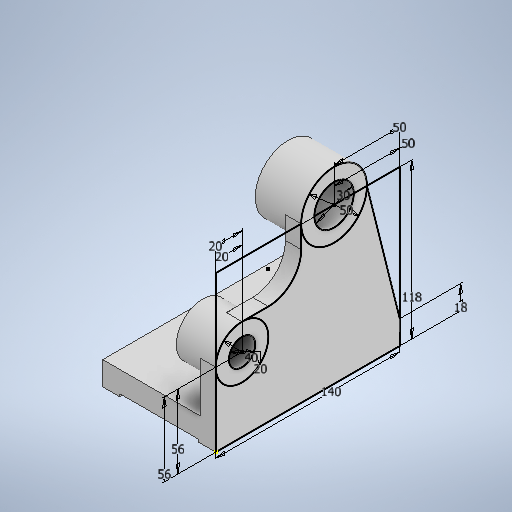
# Autodesk Inventor part: 3
Saved by Autodesk Inventor 2025.2 (Build 292293000, 293)
## iProperties
Created: 2024-12-04
Part Number: 3
Material: Generic
Document SubType Name: Modeling
Designer: hongquan
Density: 1 g/cm^3
Appearance: Default
Author: hongquan
Autodesk Inventor part; units mm, degrees
ref_plane "YZ Plane" through (0, 0, 0) normal (1, 0, 0) x (0, 1, 0)
ref_plane "XZ Plane" through (0, 0, 0) normal (0, 1, 0) x (-1, 0, 0)
ref_plane "XY Plane" through (0, 0, 0) normal (0, 0, 1) x (1, 0, 0)
sketch "Sketch1" plane through (0, 0, 0) normal (1, 0, 0) x (0, 1, 0)
  point P0 (0, 0)
sketch "Sketch2" plane through (0, 0, 0) normal (1, 0, 0) x (0, 1, 0)
  line L0 (0, 0) -> (118, 0)
  line L1 (118, 0) -> (118, -140)
  line L2 (118, -140) -> (0, -140)
  line L3 (0, -140) -> (0, 0)
  circle A0 centre (56, -20) radius 20
  circle A1 centre (56, -20) radius 10
  circle A2 centre (118, -90) radius 15
  circle A3 centre (118, -90) radius 25
  line L4 (118, -115) -> (18, -140)
  line L5 (101, -65) -> (118, -65)
  line L6 (76, -20) -> (76, -40)
  arc A4 (76, -40) -> (101, -65) centre (101, -40) ccw
  point P0 (56, 0)
  dimension "d2" = 40
  dimension "d0" = 140
  dimension "d1" = 118
  dimension "d3" = 20
  dimension "d4" = 30
  dimension "d5" = 50
  dimension "d6" = 56
  dimension "d7" = 56
  dimension "d8" = 20
  dimension "d9" = 20
  dimension "d10" = 50
  dimension "d11" = 50
  dimension "d12" = 18
  constraints: 14 end point, 4 centre point, 4 point on circle, 4 point on line, 3 tangent, 2 horizontal, 2 parallel, 1 perpendicular, 1 vertical, 4 other
  measures "d0" distance of L2.end L0.start
  measures "d1" distance of L1.end L2.end
  measures "d3" diameter of A1
  measures "d4" diameter of A2
  measures "d5" diameter of A3
  measures "d6" distance from line of L3 A1.centre
  measures "d7" distance from line of L3 point (56, -20)
  measures "d8" distance from line of L0 A1.centre
  measures "d9" distance from line of L0 point (56, -20)
  measures "d10" distance from line of L2 A2.centre
  measures "d11" distance from line of L2 A3.centre
  measures "d12" distance from line of L3 L4.end
sketch "Sketch3" plane through (0, 0, 0) normal (0, 0, 1) x (1, 0, 0)
  line L0 (0, 0) -> (-86, 0)
  line L1 (-86, 0) -> (-86, 18)
  line L2 (-86, 18) -> (0, 18)
  line L3 (0, 18) -> (0, 0)
  line L4 (-73, 2) -> (-13, 2)
  line L5 (-43, 18) -> (-43, 0)
  line L6 (-73, 2) -> (-73, 0)
  line L7 (-13, 2) -> (-13, 0)
  point P0 (-43, 2)
  dimension "d14" = 86
  dimension "d15" = 18
  dimension "d16" = 60
  dimension "d17" = 2
  constraints: 16 end point, 5 perpendicular, 3 midpoint, 3 point on line, 2 horizontal
  measures "d14" distance of L0.start L0.end
  measures "d15" distance of L0.end L1.end
  measures "d16" distance of L4.start L4.end
  measures "d17" distance between parallel lines of L0 L4
extrude "Extrusion1" add sketch "Sketch3" against normal blind 140 contours L0 L7 L4 L5 L2 L3 | L5 L4 L6 L0 L1 L2
extrude "Extrusion2" add sketch "Sketch2" against normal blind 12 contours L0 A0 L6 A4 L5 A3 L4 L2 L3
extrude "Extrusion3" add sketch "Sketch2" against normal blind 30 contours A0
extrude "Extrusion4" add sketch "Sketch2" against normal blind 35 contours A3 L1 A2 | L1 A2 A3
sketch "Sketch4" plane through (-73, 2, 0) normal (0, -1, 0) x (1, 0, 0)
  circle A0 centre (28.7142, -108.9689) radius 5
  circle A1 centre (33.7142, -71.4681) radius 5
  circle A2 centre (21.1452, -46.0088) radius 5
  line L0 (43, 0) -> (43, -40) projected
  circle A3 centre (43, -35.8595) radius 5
  point P0 (73, 0)
  dimension "d26" = 10
  dimension "d27" = 10
  dimension "d28" = 10
  dimension "d29" = 10
  constraints: 4 centre point, 1 point on line
  measures "d26" diameter of A0
  measures "d27" diameter of A1
  measures "d28" diameter of A2
  measures "d29" diameter of A3
extrude "Extrusion5" cut sketch "Sketch4" against normal blind 18
body "Solid1"
